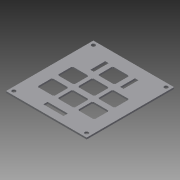
# Autodesk Inventor part: prototype
Saved by Autodesk Inventor 2015 (Build 190159000, 159)
## iProperties
Created: 2015-07-10
Part Number: prototype
Material: Generic
Document SubType Name: Modeling
Designer: Ben
Density: 1 g/cm^3
Appearance: Default
Author: Ben
Autodesk Inventor part; units mm, degrees
ref_plane "YZ Plane" through (0, 0, 0) normal (1, 0, 0) x (0, 1, 0)
ref_plane "XZ Plane" through (0, 0, 0) normal (0, 1, 0) x (-1, 0, 0)
ref_plane "XY Plane" through (0, 0, 0) normal (0, 0, 1) x (1, 0, 0)
sketch "1u" plane through (0, 0, 0) normal (0, 1, 0) x (-1, 0, 0)
  line L0 (7, 7) -> (-7, 7)
  line L1 (-7, 7) -> (-7, 6.4)
  line L2 (-7, 6.4) -> (-7.8, 6.4)
  line L3 (-7.8, 6.4) -> (-7.8, -6.4)
  line L4 (-7.8, -6.4) -> (-7, -6.4)
  line L5 (-7, -6.4) -> (-7, -7)
  line L6 (-7, -7) -> (7, -7)
  line L7 (7, -7) -> (7, -6.4)
  line L8 (7, -6.4) -> (7.8, -6.4)
  line L9 (7.8, -6.4) -> (7.8, 6.4)
  line L10 (7.8, 6.4) -> (7, 6.4)
  line L11 (7, 6.4) -> (7, 7)
  line L12 (9.525, -9.525) -> (9.525, 9.525) construction
  line L13 (9.525, 9.525) -> (-9.525, 9.525) construction
  line L14 (-9.525, 9.525) -> (-9.525, -9.525) construction
  line L15 (-9.525, -9.525) -> (9.525, -9.525) construction
  line L16 (9.525, 0) -> (7.8, 0) construction
  line L17 (-7.8, 0) -> (-9.525, 0) construction
  line L18 (0, 7) -> (0, 9.525) construction
  line L19 (0, -7) -> (0, -9.525) construction
  dimension "d0" = 12.8
  dimension "d1" = 14
  dimension "d2" = 14
  dimension "d3" = 15.6
  dimension "d4" = 19.05
  dimension "d5" = 19.05
  constraints: 40 end point, 14 perpendicular, 8 midpoint, 7 point on line, 6 collinear, 1 horizontal, 1 parallel, 1 vertical
  measures "d0" distance of L8.end L9.end
  measures "d1" distance between parallel lines of L0 L6
  measures "d2" distance of L5.end L6.end
  measures "d3" distance between parallel lines of L3 L9
  measures "d4" distance of L14.end L12.start
  measures "d5" distance of L12.start L12.end
sketch "1.25u" plane through (0, 0, 0) normal (0, 1, 0) x (-1, 0, 0)
  line L0 (7, 7) -> (-7, 7)
  line L1 (-7, 7) -> (-7, 6.4)
  line L2 (-7, 6.4) -> (-7.8, 6.4)
  line L3 (-7.8, 6.4) -> (-7.8, -6.4)
  line L4 (-7.8, -6.4) -> (-7, -6.4)
  line L5 (-7, -6.4) -> (-7, -7)
  line L6 (-7, -7) -> (7, -7)
  line L7 (7, -7) -> (7, -6.4)
  line L8 (7, -6.4) -> (7.8, -6.4)
  line L9 (7.8, -6.4) -> (7.8, 6.4)
  line L10 (7.8, 6.4) -> (7, 6.4)
  line L11 (7, 6.4) -> (7, 7)
  line L12 (11.9063, -9.525) -> (11.9063, 9.525) construction
  line L13 (11.9063, 9.525) -> (-11.9062, 9.525) construction
  line L14 (-11.9062, 9.525) -> (-11.9062, -9.525) construction
  line L15 (-11.9062, -9.525) -> (11.9063, -9.525) construction
  line L16 (11.9062, 0) -> (7.8, 0) construction
  line L17 (-7.8, 0) -> (-11.9062, 0) construction
  line L18 (0, 7) -> (0, 9.525) construction
  line L19 (0, -7) -> (0, -9.525) construction
  dimension "d45" = 12.8
  dimension "d46" = 14
  dimension "d47" = 14
  dimension "d48" = 15.6
  dimension "d49" = 23.8125
  dimension "d50" = 19.05
  constraints: 40 end point, 14 perpendicular, 8 midpoint, 7 point on line, 6 collinear, 1 horizontal, 1 parallel, 1 vertical
  measures "d45" distance of L8.end L9.end
  measures "d46" distance between parallel lines of L0 L6
  measures "d47" distance of L5.end L6.end
  measures "d48" distance between parallel lines of L3 L9
  measures "d49" distance of L14.end L12.start
  measures "d50" distance of L12.start L12.end
sketch "1.5u" plane through (0, 0, 0) normal (0, 1, 0) x (-1, 0, 0)
  line L0 (7, 7) -> (-7, 7)
  line L1 (-7, 7) -> (-7, 6.4)
  line L2 (-7, 6.4) -> (-7.8, 6.4)
  line L3 (-7.8, 6.4) -> (-7.8, -6.4)
  line L4 (-7.8, -6.4) -> (-7, -6.4)
  line L5 (-7, -6.4) -> (-7, -7)
  line L6 (-7, -7) -> (7, -7)
  line L7 (7, -7) -> (7, -6.4)
  line L8 (7, -6.4) -> (7.8, -6.4)
  line L9 (7.8, -6.4) -> (7.8, 6.4)
  line L10 (7.8, 6.4) -> (7, 6.4)
  line L11 (7, 6.4) -> (7, 7)
  line L12 (14.2875, -9.525) -> (14.2875, 9.525) construction
  line L13 (14.2875, 9.525) -> (-14.2875, 9.525) construction
  line L14 (-14.2875, 9.525) -> (-14.2875, -9.525) construction
  line L15 (-14.2875, -9.525) -> (14.2875, -9.525) construction
  line L16 (14.2875, 0) -> (7.8, 0) construction
  line L17 (-7.8, 0) -> (-14.2875, 0) construction
  line L18 (0, 7) -> (0, 9.525) construction
  line L19 (0, -7) -> (0, -9.525) construction
  dimension "d39" = 12.8
  dimension "d40" = 14
  dimension "d41" = 14
  dimension "d42" = 15.6
  dimension "d43" = 28.575
  dimension "d44" = 19.05
  constraints: 40 end point, 14 perpendicular, 8 midpoint, 7 point on line, 6 collinear, 1 horizontal, 1 parallel, 1 vertical
  measures "d39" distance of L8.end L9.end
  measures "d40" distance between parallel lines of L0 L6
  measures "d41" distance of L5.end L6.end
  measures "d42" distance between parallel lines of L3 L9
  measures "d43" distance of L14.end L12.start
  measures "d44" distance of L12.start L12.end
sketch "2u" plane through (0, 0, 0) normal (0, 1, 0) x (-1, 0, 0)
  line L0 (7, -7) -> (7, -6.4)
  line L1 (7, -6.4) -> (7.8, -6.4)
  line L2 (19.05, 0) -> (7.8, 0) construction
  line L3 (19.05, -9.525) -> (19.05, 9.525) construction
  line L4 (7.8, -6.4) -> (7.8, 6.4)
  line L5 (0, -7) -> (0, -9.525) construction
  line L6 (-7, -6.4) -> (-7, -7)
  line L7 (-7.8, 0) -> (-19.05, 0) construction
  line L8 (-7.8, -6.4) -> (-7, -6.4)
  line L9 (0, 7) -> (0, 9.525) construction
  line L10 (7, 7) -> (-7, 7)
  line L11 (-7, -7) -> (7, -7)
  line L12 (-19.05, -9.525) -> (19.05, -9.525) construction
  line L13 (19.05, 9.525) -> (-19.05, 9.525) construction
  line L14 (-19.05, 9.525) -> (-19.05, -9.525) construction
  line L15 (-7, 7) -> (-7, 6.4)
  line L16 (-7, 6.4) -> (-7.8, 6.4)
  line L17 (-7.8, 6.4) -> (-7.8, -6.4)
  line L18 (7, 6.4) -> (7, 7)
  line L19 (7.8, 6.4) -> (7, 6.4)
  line L20 (15.6, -6.24) -> (15.6, 7.76)
  line L21 (15.6, 7.76) -> (12.4, 7.76)
  line L22 (12.4, 7.76) -> (12.4, -6.24)
  line L23 (12.4, -6.24) -> (15.6, -6.24)
  line L24 (14, -6.24) -> (14, 7.76) construction
  line L25 (15.6, 0.76) -> (12.4, 0.76) construction
  line L26 (-12.4, 7.76) -> (-12.4, -6.24)
  line L27 (-12.4, -6.24) -> (-15.6, -6.24)
  line L28 (-15.6, -6.24) -> (-15.6, 7.76)
  line L29 (-15.6, 7.76) -> (-12.4, 7.76)
  line L30 (-14, -6.24) -> (-14, 7.76) construction
  line L31 (-15.6, 0.76) -> (-12.4, 0.76) construction
  dimension "d28" = 12.8
  dimension "d29" = 14
  dimension "d30" = 14
  dimension "d31" = 15.6
  dimension "d32" = 38.1
  dimension "d33" = 19.05
  dimension "d34" = 3.2
  dimension "d35" = 14
  dimension "d36" = 14
  dimension "d37" = 0.76
  constraints: 64 end point, 17 perpendicular, 12 midpoint, 8 symmetric about line, 7 point on line, 6 collinear, 2 vertical, 1 horizontal, 1 parallel
  measures "d28" distance of L4.start L4.end
  measures "d29" distance between parallel lines of L10 L11
  measures "d30" distance of L11.start L0.start
  measures "d31" distance between parallel lines of L17 L4
  measures "d32" distance of L12.start L3.start
  measures "d33" distance of L3.start L3.end
  measures "d34" distance of L22.end L20.start
  measures "d35" distance of L20.start L21.start
  measures "d36" distance between parallel lines of L5 L24
  measures "d37" distance between parallel lines of L25 L2
sketch "Sketch11" plane through (0, 0, 0) normal (0, 1, 0) x (1, 0, 0)
  line L0 (10.7522, 7.1342) -> (-3.2478, 7.1342)
  line L1 (-3.2478, 7.1342) -> (-3.2478, 6.5342)
  line L2 (-3.2478, 6.5342) -> (-4.0478, 6.5342)
  line L3 (-4.0478, 6.5342) -> (-4.0478, -6.2658)
  line L4 (-4.0478, -6.2658) -> (-3.2478, -6.2658)
  line L5 (-3.2478, -6.2658) -> (-3.2478, -6.8658)
  line L6 (-3.2478, -6.8658) -> (10.7522, -6.8658)
  line L7 (10.7522, -6.8658) -> (10.7522, -6.2658)
  line L8 (10.7522, -6.2658) -> (11.5522, -6.2658)
  line L9 (11.5522, -6.2658) -> (11.5522, 6.5342)
  line L10 (11.5522, 6.5342) -> (10.7522, 6.5342)
  line L11 (10.7522, 6.5342) -> (10.7522, 7.1342)
  line L12 (13.2772, -9.3908) -> (13.2772, 9.6592) construction
  line L13 (13.2772, 9.6592) -> (-5.7728, 9.6592) construction
  line L14 (-5.7728, 9.6592) -> (-5.7728, -9.3908) construction
  line L15 (-5.7728, -9.3908) -> (13.2772, -9.3908) construction
  line L16 (13.2772, 0.1342) -> (11.5522, 0.1342) construction
  line L17 (-4.0478, 0.1342) -> (-5.7728, 0.1342) construction
  line L18 (3.7522, 7.1342) -> (3.7522, 9.6592) construction
  line L19 (3.7522, -6.8658) -> (3.7522, -9.3908) construction
  line L20 (29.8022, 7.1342) -> (15.8022, 7.1342)
  line L21 (15.8022, 7.1342) -> (15.8022, 6.5342)
  line L22 (15.8022, 6.5342) -> (15.0022, 6.5342)
  line L23 (15.0022, 6.5342) -> (15.0022, -6.2658)
  line L24 (15.0022, -6.2658) -> (15.8022, -6.2658)
  line L25 (15.8022, -6.2658) -> (15.8022, -6.8658)
  line L26 (15.8022, -6.8658) -> (29.8022, -6.8658)
  line L27 (29.8022, -6.8658) -> (29.8022, -6.2658)
  line L28 (29.8022, -6.2658) -> (30.6022, -6.2658)
  line L29 (30.6022, -6.2658) -> (30.6022, 6.5342)
  line L30 (30.6022, 6.5342) -> (29.8022, 6.5342)
  line L31 (29.8022, 6.5342) -> (29.8022, 7.1342)
  line L32 (32.3272, -9.3908) -> (32.3272, 9.6592) construction
  line L33 (32.3272, 9.6592) -> (13.2772, 9.6592) construction
  line L34 (13.2772, 9.6592) -> (13.2772, -9.3908) construction
  line L35 (13.2772, -9.3908) -> (32.3272, -9.3908) construction
  line L36 (32.3272, 0.1342) -> (30.6022, 0.1342) construction
  line L37 (15.0022, 0.1342) -> (13.2772, 0.1342) construction
  line L38 (22.8022, 7.1342) -> (22.8022, 9.6592) construction
  line L39 (22.8022, -6.8658) -> (22.8022, -9.3908) construction
  line L40 (48.8522, 7.1342) -> (34.8522, 7.1342)
  line L41 (34.8522, 7.1342) -> (34.8522, 6.5342)
  line L42 (34.8522, 6.5342) -> (34.0522, 6.5342)
  line L43 (34.0522, 6.5342) -> (34.0522, -6.2658)
  line L44 (34.0522, -6.2658) -> (34.8522, -6.2658)
  line L45 (34.8522, -6.2658) -> (34.8522, -6.8658)
  line L46 (34.8522, -6.8658) -> (48.8522, -6.8658)
  line L47 (48.8522, -6.8658) -> (48.8522, -6.2658)
  line L48 (48.8522, -6.2658) -> (49.6522, -6.2658)
  line L49 (49.6522, -6.2658) -> (49.6522, 6.5342)
  line L50 (49.6522, 6.5342) -> (48.8522, 6.5342)
  line L51 (48.8522, 6.5342) -> (48.8522, 7.1342)
  line L52 (51.3772, -9.3908) -> (51.3772, 9.6592) construction
  line L53 (51.3772, 9.6592) -> (32.3272, 9.6592) construction
  line L54 (32.3272, 9.6592) -> (32.3272, -9.3908) construction
  line L55 (32.3272, -9.3908) -> (51.3772, -9.3908) construction
  line L56 (51.3772, 0.1342) -> (49.6522, 0.1342) construction
  line L57 (34.0522, 0.1342) -> (32.3272, 0.1342) construction
  line L58 (41.8522, 7.1342) -> (41.8522, 9.6592) construction
  line L59 (41.8522, -6.8658) -> (41.8522, -9.3908) construction
  line L60 (10.7522, -11.9158) -> (-3.2478, -11.9158)
  line L61 (-3.2478, -11.9158) -> (-3.2478, -12.5158)
  line L62 (-3.2478, -12.5158) -> (-4.0478, -12.5158)
  line L63 (-4.0478, -12.5158) -> (-4.0478, -25.3158)
  line L64 (-4.0478, -25.3158) -> (-3.2478, -25.3158)
  line L65 (-3.2478, -25.3158) -> (-3.2478, -25.9158)
  line L66 (-3.2478, -25.9158) -> (10.7522, -25.9158)
  line L67 (10.7522, -25.9158) -> (10.7522, -25.3158)
  line L68 (10.7522, -25.3158) -> (11.5522, -25.3158)
  line L69 (11.5522, -25.3158) -> (11.5522, -12.5158)
  line L70 (11.5522, -12.5158) -> (10.7522, -12.5158)
  line L71 (10.7522, -12.5158) -> (10.7522, -11.9158)
  line L72 (13.2772, -28.4408) -> (13.2772, -9.3908) construction
  line L73 (13.2772, -9.3908) -> (-5.7728, -9.3908) construction
  line L74 (-5.7728, -9.3908) -> (-5.7728, -28.4408) construction
  line L75 (-5.7728, -28.4408) -> (13.2772, -28.4408) construction
  line L76 (13.2772, -18.9158) -> (11.5522, -18.9158) construction
  line L77 (-4.0478, -18.9158) -> (-5.7728, -18.9158) construction
  line L78 (3.7522, -11.9158) -> (3.7522, -9.3908) construction
  line L79 (3.7522, -25.9158) -> (3.7522, -28.4408) construction
  line L80 (29.8022, -11.9158) -> (15.8022, -11.9158)
  line L81 (15.8022, -11.9158) -> (15.8022, -12.5158)
  line L82 (15.8022, -12.5158) -> (15.0022, -12.5158)
  line L83 (15.0022, -12.5158) -> (15.0022, -25.3158)
  line L84 (15.0022, -25.3158) -> (15.8022, -25.3158)
  line L85 (15.8022, -25.3158) -> (15.8022, -25.9158)
  line L86 (15.8022, -25.9158) -> (29.8022, -25.9158)
  line L87 (29.8022, -25.9158) -> (29.8022, -25.3158)
  line L88 (29.8022, -25.3158) -> (30.6022, -25.3158)
  line L89 (30.6022, -25.3158) -> (30.6022, -12.5158)
  line L90 (30.6022, -12.5158) -> (29.8022, -12.5158)
  line L91 (29.8022, -12.5158) -> (29.8022, -11.9158)
  line L92 (32.3272, -28.4408) -> (32.3272, -9.3908) construction
  line L93 (32.3272, -9.3908) -> (13.2772, -9.3908) construction
  line L94 (13.2772, -9.3908) -> (13.2772, -28.4408) construction
  line L95 (13.2772, -28.4408) -> (32.3272, -28.4408) construction
  line L96 (32.3272, -18.9158) -> (30.6022, -18.9158) construction
  line L97 (15.0022, -18.9158) -> (13.2772, -18.9158) construction
  line L98 (22.8022, -11.9158) -> (22.8022, -9.3908) construction
  line L99 (22.8022, -25.9158) -> (22.8022, -28.4408) construction
  line L100 (48.8522, -11.9158) -> (34.8522, -11.9158)
  line L101 (34.8522, -11.9158) -> (34.8522, -12.5158)
  line L102 (34.8522, -12.5158) -> (34.0522, -12.5158)
  line L103 (34.0522, -12.5158) -> (34.0522, -25.3158)
  line L104 (34.0522, -25.3158) -> (34.8522, -25.3158)
  line L105 (34.8522, -25.3158) -> (34.8522, -25.9158)
  line L106 (34.8522, -25.9158) -> (48.8522, -25.9158)
  line L107 (48.8522, -25.9158) -> (48.8522, -25.3158)
  line L108 (48.8522, -25.3158) -> (49.6522, -25.3158)
  line L109 (49.6522, -25.3158) -> (49.6522, -12.5158)
  line L110 (49.6522, -12.5158) -> (48.8522, -12.5158)
  line L111 (48.8522, -12.5158) -> (48.8522, -11.9158)
  line L112 (51.3772, -28.4408) -> (51.3772, -9.3908) construction
  line L113 (51.3772, -9.3908) -> (32.3272, -9.3908) construction
  line L114 (32.3272, -9.3908) -> (32.3272, -28.4408) construction
  line L115 (32.3272, -28.4408) -> (51.3772, -28.4408) construction
  line L116 (51.3772, -18.9158) -> (49.6522, -18.9158) construction
  line L117 (34.0522, -18.9158) -> (32.3272, -18.9158) construction
  line L118 (41.8522, -11.9158) -> (41.8522, -9.3908) construction
  line L119 (41.8522, -25.9158) -> (41.8522, -28.4408) construction
  line L120 (41.8522, 19.1842) -> (30.6022, 19.1842) construction
  line L121 (30.6022, 12.7842) -> (30.6022, 25.5842)
  line L122 (41.8522, 9.6592) -> (41.8522, 28.7092) construction
  line L123 (29.8022, 12.7842) -> (30.6022, 12.7842)
  line L124 (29.8022, 12.1842) -> (29.8022, 12.7842)
  line L125 (3.7522, 9.6592) -> (41.8522, 9.6592) construction
  line L126 (41.8522, 28.7092) -> (3.7522, 28.7092) construction
  line L127 (22.8022, 26.1842) -> (22.8022, 28.7092) construction
  line L128 (22.8022, 12.1842) -> (22.8022, 9.6592) construction
  line L129 (15.8022, 12.1842) -> (29.8022, 12.1842)
  line L130 (29.8022, 26.1842) -> (15.8022, 26.1842)
  line L131 (15.8022, 12.7842) -> (15.8022, 12.1842)
  line L132 (15.0022, 12.7842) -> (15.8022, 12.7842)
  line L133 (15.0022, 25.5842) -> (15.0022, 12.7842)
  line L134 (15.8022, 26.1842) -> (15.8022, 25.5842)
  line L135 (15.8022, 25.5842) -> (15.0022, 25.5842)
  line L136 (7.2022, 26.9442) -> (10.4022, 26.9442)
  line L137 (29.8022, 25.5842) -> (29.8022, 26.1842)
  line L138 (30.6022, 25.5842) -> (29.8022, 25.5842)
  line L139 (38.4022, 26.9442) -> (35.2022, 26.9442)
  line L140 (35.2022, 26.9442) -> (35.2022, 12.9442)
  line L141 (36.8022, 12.9442) -> (36.8022, 26.9442) construction
  line L142 (38.4022, 12.9442) -> (38.4022, 26.9442)
  line L143 (38.4022, 19.9442) -> (35.2022, 19.9442) construction
  line L144 (35.2022, 12.9442) -> (38.4022, 12.9442)
  line L145 (7.2022, 19.9442) -> (10.4022, 19.9442) construction
  line L146 (10.4022, 26.9442) -> (10.4022, 12.9442)
  line L147 (15.0022, 19.1842) -> (3.7522, 19.1842) construction
  line L148 (8.8022, 12.9442) -> (8.8022, 26.9442) construction
  line L149 (7.2022, 12.9442) -> (7.2022, 26.9442)
  line L150 (3.7522, 28.7092) -> (3.7522, 9.6592) construction
  line L151 (10.4022, 12.9442) -> (7.2022, 12.9442)
  line L152 (-7.7278, 30.6642) -> (53.3322, 30.6642) construction
  line L153 (53.3322, 30.6642) -> (53.3322, -36.7458) construction
  line L154 (53.3322, -36.7458) -> (-7.7278, -36.7458) construction
  line L155 (-7.7278, -36.7458) -> (-7.7278, 30.6642) construction
  line L156 (-7.7278, -3.0408) -> (-5.7728, -3.0408) construction
  line L157 (53.3322, -3.0408) -> (51.3772, -3.0408) construction
  line L158 (22.8022, 30.6642) -> (22.8022, 28.7092) construction
  line L159 (-15.2278, 38.1642) -> (60.8322, 38.1642)
  line L160 (60.8322, 38.1642) -> (60.8322, -44.2458)
  line L161 (60.8322, -44.2458) -> (-15.2278, -44.2458)
  line L162 (-15.2278, -44.2458) -> (-15.2278, 38.1642)
  line L163 (22.8022, 38.1642) -> (22.8022, 30.6642) construction
  line L164 (60.8322, -3.0408) -> (53.3322, -3.0408) construction
  line L165 (-15.2278, -3.0408) -> (-7.7278, -3.0408) construction
  line L166 (22.8022, -44.2458) -> (22.8022, -36.7458) construction
  line L167 (13.2772, -33.4758) -> (32.3272, -33.4758)
  line L168 (32.3272, -33.4758) -> (32.3272, -37.4758)
  line L169 (32.3272, -37.4758) -> (13.2772, -37.4758)
  line L170 (13.2772, -37.4758) -> (13.2772, -33.4758)
  line L171 (13.2772, -35.4758) -> (32.3272, -35.4758) construction
  line L172 (-11.4778, 34.4142) -> (57.0822, 34.4142) construction
  line L173 (57.0822, 34.4142) -> (57.0822, -40.4958) construction
  line L174 (57.0822, -40.4958) -> (-11.4778, -40.4958) construction
  line L175 (-11.4778, -40.4958) -> (-11.4778, 34.4142) construction
  circle A0 centre (-11.4778, 34.4142) radius 1.75
  circle A1 centre (57.0822, 34.4142) radius 1.75
  circle A2 centre (57.0822, -40.4958) radius 1.75
  circle A3 centre (-11.4778, -40.4958) radius 1.75
  line L176 (-7.7278, 38.1642) -> (-7.7278, 34.4142) construction
  line L177 (-7.7278, 30.6642) -> (-7.7278, 34.4142) construction
  line L178 (-7.7278, 30.6642) -> (-11.4778, 30.6642) construction
  line L179 (-11.4778, 30.6642) -> (-15.2278, 30.6642) construction
  line L180 (53.3322, 30.6642) -> (57.0822, 30.6642) construction
  line L181 (57.0822, 30.6642) -> (60.8322, 30.6642) construction
  line L182 (53.3322, -36.7458) -> (53.3322, -40.4958) construction
  line L183 (53.3322, -40.4958) -> (53.3322, -44.2458) construction
  point P0 (0, 0)
  dimension "d298" = 12.8
  dimension "d299" = 14
  dimension "d300" = 14
  dimension "d301" = 15.6
  dimension "d302" = 19.05
  dimension "d303" = 19.05
  dimension "d306" = 19.05
  dimension "d309" = 19.05
  dimension "d312" = 12.8
  dimension "d313" = 14
  dimension "d314" = 14
  dimension "d315" = 15.6
  dimension "d316" = 38.1
  dimension "d317" = 19.05
  dimension "d318" = 3.2
  dimension "d319" = 14
  dimension "d320" = 14
  dimension "d321" = 0.76
  dimension "d323" = 61.06
  dimension "d324" = 67.41
  dimension "d325" = 7.5
  dimension "d326" = 1.27
  dimension "d327" = 4
  dimension "d328" = 3.5
  dimension "d329" = 3.5
  dimension "d330" = 3.5
  dimension "d331" = 3.5
  constraints: 368 end point, 68 point on line, 44 perpendicular, 33 midpoint, 16 equal length, 10 collinear, 10 parallel, 8 symmetric about line, 7 horizontal, 4 centre point, 4 coincident, 4 vertical, 218 other
  measures "d298" distance of L8.end L9.end
  measures "d299" distance between parallel lines of L0 L6
  measures "d300" distance of L5.end L6.end
  measures "d301" distance between parallel lines of L3 L9
  measures "d302" distance of L14.end L12.start
  measures "d303" distance of L12.start L12.end
  measures "d306" distance of L10.end L31.start
  measures "d309" distance of L10.end L71.start
  measures "d312" distance of L121.start L121.end
  measures "d313" distance between parallel lines of L130 L129
  measures "d314" distance of L129.start L124.start
  measures "d315" distance between parallel lines of L133 L121
  measures "d316" distance of L125.start L122.start
  measures "d317" distance of L122.start L122.end
  measures "d318" distance of L140.end L142.start
  measures "d319" distance of L142.start L139.start
  measures "d320" distance between parallel lines of L128 L141
  measures "d321" distance between parallel lines of L143 L120
  measures "d323" distance of L153.end L154.end
  measures "d324" distance of L152.end L153.end
  measures "d325" distance of L163.start L163.end
  measures "d326" distance between parallel lines of L154 L171
  measures "d327" distance between parallel lines of L169 L167
  measures "d328" diameter of A0
  measures "d329" diameter of A1
  measures "d330" diameter of A2
  measures "d331" diameter of A3
extrude "Extrusion3" add sketch "Sketch11" along normal blind 1.5
body "Solid3"
